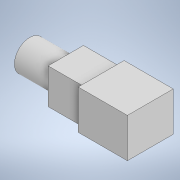
# Autodesk Inventor part: Plug
Saved by Autodesk Inventor 2020 (Build 240168000, 168)
## iProperties
Created: 2020-01-26
Part Number: Plug
Material: Generic
Document SubType Name: Modeling
Designer: holtat
Density: 1 g/cm^3
Appearance: Default
Author: holtat
Autodesk Inventor part; units mm, degrees
ref_plane "YZ Plane" through (0, 0, 0) normal (1, 0, 0) x (0, 1, 0)
ref_plane "XZ Plane" through (0, 0, 0) normal (0, 1, 0) x (-1, 0, 0)
ref_plane "XY Plane" through (0, 0, 0) normal (0, 0, 1) x (1, 0, 0)
sketch "Sketch1" plane through (0, 0, 0) normal (0, 1, 0) x (-1, 0, 0)
  line L0 (7.9502, -7.4168) -> (-7.9502, -7.4168)
  line L1 (-7.9502, -7.4168) -> (-7.9502, 7.4168)
  line L2 (-7.9502, 7.4168) -> (7.9502, 7.4168)
  line L3 (7.9502, 7.4168) -> (7.9502, -7.4168)
  point P0 (0, 0)
  point P1 (7.9502, 0)
  point P2 (0, -7.4168)
  dimension "d0" = 14.8336
  dimension "d1" = 15.9004
  constraints: 8 end point, 2 midpoint, 2 parallel, 1 horizontal, 1 horizontal alignment, 1 perpendicular, 1 vertical alignment
  measures "d0" distance of L2.end L0.start
  measures "d1" distance between parallel lines of L3 L1
extrude "Extrusion1" add sketch "Sketch1" along normal mid plane 12.7
sketch "Sketch2" plane through (-7.9502, -6.35, 7.4168) normal (-1, 0, 0) x (0, 0, 1)
  line L0 (0, 0) -> (0, 12.7) projected
  line L1 (-14.8336, 12.7) -> (0, 12.7) projected
  line L2 (-14.8336, 0) -> (-14.8336, 12.7) projected
  line L3 (0, 0) -> (-14.8336, 0) projected
  line L4 (-13.1318, 12.065) -> (-1.7018, 12.065)
  line L5 (-1.7018, 12.065) -> (-1.7018, 0.635)
  line L6 (-1.7018, 0.635) -> (-13.1318, 0.635)
  line L7 (-13.1318, 0.635) -> (-13.1318, 12.065)
  point P0 (-7.4168, 6.35)
  point P1 (-13.1318, 6.35)
  point P2 (-7.4168, 12.065)
  dimension "d11" = 11.43
  dimension "d12" = 11.43
  constraints: 8 end point, 2 midpoint, 2 parallel, 1 horizontal, 1 horizontal alignment, 1 perpendicular, 1 vertical alignment
  measures "d11" distance between parallel lines of L5 L7
  measures "d12" distance between parallel lines of L6 L4
extrude "Extrusion2" add sketch "Sketch2" along normal blind 11.43 contours L4 L5 L6 L7
sketch "Sketch3" plane through (-19.3802, -6.35, 7.4168) normal (-1, 0, 0) x (0, 0, 1)
  circle A0 centre (-7.4168, 6.35) radius 4.953
  dimension "d10" = 9.906
  constraints: 1 centre point, 1 coincident
  measures "d10" diameter of A0
extrude "Extrusion3" add sketch "Sketch3" along normal blind 11.684
equation "\"d12\" = d11"
body "Solid1"
